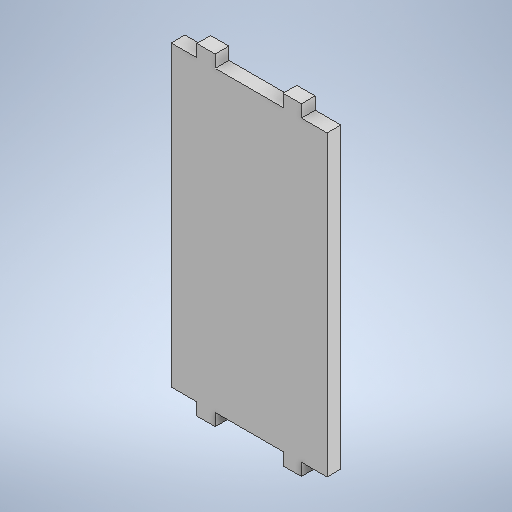
# Autodesk Inventor part: carcasa_piezaLateral_ruedas
Saved by Autodesk Inventor 2025.2 (Build 292293000, 293)
## iProperties
Created: 2025-09-08
Part Number: carcasa_piezaLateral_ruedas
Material: Generic
Document SubType Name: Modeling
Designer: brene
Density: 1 g/cm^3
Appearance: Default
Author: brene
Autodesk Inventor part; units mm, degrees
ref_plane "YZ Plane" through (0, 0, 0) normal (1, 0, 0) x (0, 1, 0)
ref_plane "XZ Plane" through (0, 0, 0) normal (0, 1, 0) x (-1, 0, 0)
ref_plane "XY Plane" through (0, 0, 0) normal (0, 0, 1) x (1, 0, 0)
sketch "Sketch1" plane through (0, 0, 0) normal (0, 0, 1) x (1, 0, 0)
  line L0 (0, 0) -> (34, 0)
  line L1 (34, 0) -> (34, 65)
  line L2 (34, 65) -> (0, 65)
  line L3 (0, 65) -> (0, 0)
  dimension "d0" = 34
  dimension "d1" = 65
  dimension "d2" = 34
  constraints: 8 end point, 2 perpendicular, 1 horizontal
  measures "d0" distance of L0.start L0.end
  measures "d1" distance of L0.end L1.end
  measures "d2" distance of L1.end L2.end
extrude "Extrusion1" add sketch "Sketch1" along normal blind 3
sketch "Sketch2" plane through (0, 0, 0) normal (0, -1, 0) x (1, 0, 0)
  point P0 (0, 0)
sketch "Sketch3" plane through (0, 0, 0) normal (0, -1, 0) x (1, 0, 0)
  line L0 (0, 0) -> (0, 3) projected
  line L1 (0, 1.5) -> (34, 1.5)
  line L2 (34, 0) -> (34, 3) projected
  line L3 (17, 1.5) -> (9.597, 1.5)
  line L4 (9.597, 1.5) -> (9.597, 3)
  line L5 (9.597, 3) -> (5.597, 3)
  line L6 (5.597, 3) -> (5.597, 0)
  line L7 (5.597, 0) -> (9.597, 0)
  line L8 (9.597, 0) -> (9.597, 1.5)
  line L9 (17, 1.5) -> (24.403, 1.5)
  line L10 (24.403, 1.5) -> (24.403, 3)
  line L11 (24.403, 3) -> (28.403, 3)
  line L12 (28.403, 3) -> (28.403, 0)
  line L13 (28.403, 0) -> (24.403, 0)
  line L14 (24.403, 0) -> (24.403, 1.5)
  dimension "d5" = 7.403
  dimension "d6" = 1.5
  dimension "d7" = 4
  dimension "d10" = 4
  dimension "d11" = 7.403
  dimension "d12" = 1.5
  dimension "d13" = 4
  dimension "d14" = 3
  dimension "d15" = 4
  constraints: 26 end point, 5 perpendicular, 4 point on line, 3 midpoint, 2 vertical
  measures "d5" distance of L3.start L3.end
  measures "d6" distance of L3.end L4.end
  measures "d7" distance of L4.end L5.end
  measures "d10" distance of L6.end L7.end
  measures "d11" distance of L3.start L9.end
  measures "d12" distance of L9.end L10.end
  measures "d13" distance of L10.end L11.end
  measures "d14" distance of L11.end L12.end
  measures "d15" distance of L12.end L13.end
extrude "Extrusion2" add sketch "Sketch3" along normal blind 2.7
extrude "Extrusion3" add sketch "Sketch3" against normal blind 2.7 from surface at -65
body "Solid1"
